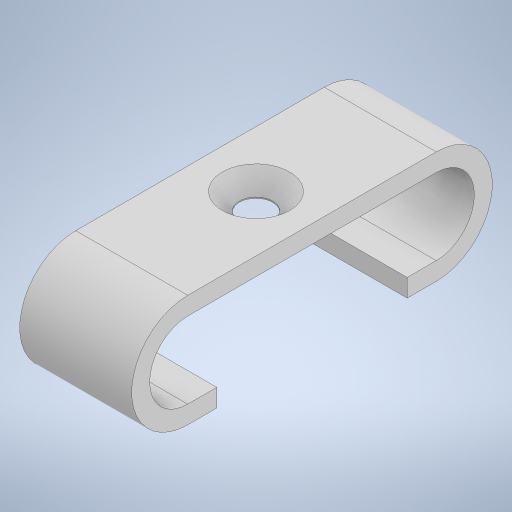
# Autodesk Inventor part: klips
Saved by Autodesk Inventor 2023.4 (Build 274418000, 418)
## iProperties
Created: 2024-08-08
Part Number: klips
Material: Generic
Document SubType Name: Modeling
Designer: komputer
Density: 1 g/cm^3
Appearance: Default
Author: komputer
Autodesk Inventor part; units mm, degrees
ref_plane "YZ Plane" through (0, 0, 0) normal (1, 0, 0) x (0, 1, 0)
ref_plane "XZ Plane" through (0, 0, 0) normal (0, 1, 0) x (-1, 0, 0)
ref_plane "XY Plane" through (0, 0, 0) normal (0, 0, 1) x (1, 0, 0)
sketch "Sketch1" plane through (0, 0, 0) normal (1, 0, 0) x (0, 1, 0)
  line L0 (-7.4638, 10.773) -> (-7.4638, 13.3671)
  line L1 (-0.652, 13.3671) -> (-0.652, 10.773)
  arc A0 (-0.652, 13.3671) -> (-7.4638, 13.3671) centre (-4.0579, 13.3671) ccw
  line L2 (0.948, 10.773) -> (0.948, 13.3671)
  arc A1 (0.948, 13.3671) -> (-9.0638, 13.3671) centre (-4.0579, 13.3671) ccw
  line L3 (-9.0638, 13.3671) -> (-9.0638, 10.773)
  line L4 (-9.0638, 10.773) -> (-7.4638, 10.773)
  line L5 (-0.652, 10.773) -> (-0.652, -6.227)
  line L6 (-4.0579, 16.773) -> (-4.0579, 10.773)
  line L7 (0.948, 10.773) -> (0.948, -6.227)
  line L8 (-0.652, 2.273) -> (-9.3077, 2.273)
  line L9 (-7.4638, -6.227) -> (-7.4638, -8.8211)
  line L10 (-0.652, -8.8211) -> (-0.652, -6.227)
  arc A2 (-7.4638, -8.8211) -> (-0.652, -8.8211) centre (-4.0579, -8.8211) ccw
  line L11 (0.948, -6.227) -> (0.948, -8.8211)
  arc A3 (-9.0638, -8.8211) -> (0.948, -8.8211) centre (-4.0579, -8.8211) ccw
  line L12 (-9.0638, -8.8211) -> (-9.0638, -6.227)
  line L13 (0.948, -6.227) -> (0.948, 10.773)
  line L14 (-9.0638, -6.227) -> (-7.4638, -6.227)
  point P0 (0, 0)
  point P1 (0.948, -6.227)
  dimension "d3" = 1.6
  dimension "d4" = 17
  dimension "d5" = 6
  constraints: 30 end point, 9 point on circle, 9 symmetric about line, 5 vertical, 4 centre point, 3 horizontal, 3 horizontal alignment, 2 tangent, 1 midpoint, 4 other
  measures "d3" distance between parallel lines of L1 L2
  measures "d4" distance of L1.end L5.end
  measures "d5" distance of L6.start L6.end
extrude "Extrusion1" add sketch "Sketch1" along normal blind 10
sketch "Sketch2" plane through (0, 0.948, 13.3671) normal (0, 1, 0) x (1, 0, 0)
  line L0 (0, 22.1882) -> (0, 0) projected
  line L1 (0, 0) -> (10, 0) projected
  line L2 (10, 22.1882) -> (10, 0) projected
  line L3 (0, 22.1882) -> (10, 22.1882) projected
  point P0 (0, 13.3671)
  point P1 (5, 11.0941)
  point P2 (0, 11.0941)
  point P3 (5, 0)
  constraints: 2 midpoint, 1 horizontal alignment, 1 vertical alignment
hole "Hole1" at (5, 0.948, 2.273) direction (0, -1, 0) diameter 3 end through all countersink diameter 6 countersink angle 90
body "Solid1"
